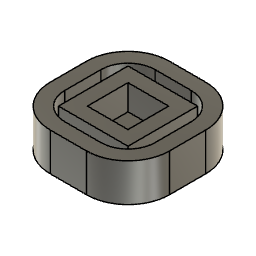
Pulsador v6 (Autodesk Fusion 360 design; units mm, degrees)
Autodesk Fusion 360 part; units mm, degrees
sketch "Boceto1" plane through (0, 0, 0) normal (0, 0, 1) x (1, 0, 0)
  line L0 (2, 5) -> (-2, 5)
  line L1 (-5, 2) -> (-5, -2)
  line L2 (-2, -5) -> (2, -5)
  line L3 (5, -2) -> (5, 2)
  line L4 (5, 5) -> (-5, -5) construction
  line L5 (-5, 5) -> (5, -5) construction
  line L6 (2.25, -2.25) -> (-2.25, -2.25)
  line L7 (-2.25, -2.25) -> (-2.25, 2.25)
  line L8 (-2.25, 2.25) -> (2.25, 2.25)
  line L9 (2.25, 2.25) -> (2.25, -2.25)
  line L10 (2.25, -2.25) -> (-2.25, 2.25) construction
  line L11 (-2.25, -2.25) -> (2.25, 2.25) construction
  line L12 (3.85, -3.85) -> (-3.85, -3.85)
  line L13 (-3.85, -3.85) -> (-3.85, 3.85)
  line L14 (-3.85, 3.85) -> (3.85, 3.85)
  line L15 (3.85, 3.85) -> (3.85, -3.85)
  arc A0 (-2, 5) -> (-5, 2) centre (-2, 2) ccw
  arc A1 (5, 2) -> (2, 5) centre (2, 2) ccw
  arc A2 (2, -5) -> (5, -2) centre (2, -2) ccw
  arc A3 (-5, -2) -> (-2, -5) centre (-2, -2) ccw
  arc A4 (-6.6, -2) -> (-2, -6.6) centre (-2, -2) ccw
  line L16 (-2, -6.6) -> (2, -6.6)
  arc A5 (2, -6.6) -> (6.6, -2) centre (2, -2) ccw
  line L17 (6.6, -2) -> (6.6, 2)
  arc A6 (6.6, 2) -> (2, 6.6) centre (2, 2) ccw
  line L18 (2, 6.6) -> (-2, 6.6)
  arc A7 (-2, 6.6) -> (-6.6, 2) centre (-2, 2) ccw
  line L19 (-6.6, 2) -> (-6.6, -2)
  dimension "d3" = 10
  dimension "d4" = 10
  dimension "d5" = 4.5
  dimension "d6" = 4.5
  dimension "d7" = -1.6
  dimension "d8" = 3
  dimension "d9" = 1.6
  constraint horizontal L0
  constraint perpendicular L0 L1
  constraint parallel L0 L2
  constraint parallel L1 L3
  constraint coincident L4 origin
  constraint coincident L5 origin
  constraint horizontal L6
  constraint perpendicular L6 L7
  constraint parallel L6 L8
  constraint parallel L7 L9
  constraint coincident L10 origin
  constraint coincident L11 origin
  constraint coincident L5.start L1
  constraint coincident L5.start L0
  constraint tangent L1 A0
  constraint tangent L0 A0
  constraint coincident L4.start L0
  constraint coincident L4.start L3
  constraint tangent L0 A1
  constraint tangent L3 A1
  constraint equal A0 A1
  constraint coincident L5.end L3
  constraint coincident L5.end L2
  constraint tangent L3 A2
  constraint tangent L2 A2
  constraint equal A0 A2
  constraint coincident L4.end L2
  constraint coincident L4.end L1
  constraint tangent L2 A3
  constraint tangent L1 A3
  constraint equal A0 A3
  measures "d3" distance of L4.end L5.end
  measures "d4" distance of L5.start L4.end
  measures "d5" distance of L7.end L8.end
  measures "d6" distance of L6.end L7.end
  measures "d8" radius of A0
extrude "Extruir1" add sketch "Boceto1" along normal blind 1.4 contours L0 L1 L2 L3 A0 A1 A2 A3 | L6 L7 L8 L9 | L12 L13 L14 L15 | A4 L16 A5 L17 A6 L18 A7 L19
extrude "Extruir2" add sketch "Boceto1" along normal blind 2.8 from surface at 1.4 contours L12 L13 L14 L15
extrude "Extruir3" add sketch "Boceto1" along normal up to surface (2.8 mm away) from surface at 1.4 contours A4 L16 A5 L17 A6 L18 A7 L19
named bodies: "Pulsador"
